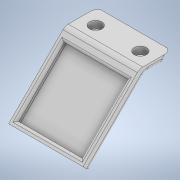
# Autodesk Inventor part: Держатель GPS
Saved by Autodesk Inventor 2022 (Build 260153000, 153)
## iProperties
Created: 2022-05-03
Part Number: Держатель GPS
Material: Типовые
Document SubType Name: Modeling
Designer: Кочетов.А.И.
Density: 1 g/cm^3
Appearance: По умолчанию
Author: Кочетов.А.И.
Autodesk Inventor part; units mm, degrees
ref_plane "YZ Plane" through (0, 0, 0) normal (1, 0, 0) x (0, 1, 0)
ref_plane "XZ Plane" through (0, 0, 0) normal (0, 1, 0) x (-1, 0, 0)
sketch "Эскиз4" plane through (0, 0, 0) normal (0, 1, 0) x (-1, 0, 0)
  line L0 (15, 10) -> (-15, 10)
  line L1 (-15, 10) -> (-15, -10)
  line L2 (-15, -10) -> (15, -10)
  line L3 (15, -10) -> (15, 10)
  line L4 (15, 10) -> (-15, -10) construction
  line L5 (-15, 10) -> (15, -10) construction
  line L6 (15, 0) -> (-15, 0) construction
  line L7 (15, 0) -> (-15, 0)
  point P0 (0, 0)
  dimension "d13" = 30
  dimension "d32" = 20
  constraints: 16 end point, 4 midpoint, 2 parallel, 2 perpendicular, 1 horizontal
  measures "d13" distance of L1.end L2.end
  measures "d32" distance of L0.end L1.end
extrude "Выдавливание4" add sketch "Эскиз4" along normal blind 3 contours L3 L2 L1 L7
ref_plane "РабПлоскость2" through (-15, 0, 0) normal (0, -0.7071068, -0.7071068) x (1, 0, 0)
sketch "Эскиз5" plane through (-15, 0, 0) normal (0, 0, 1) x (1, 0, 0)
  line L0 (0, 0) -> (30, 0) projected
  line L1 (30, 0) -> (30, 3) projected
  line L2 (0, 3) -> (30, 3) projected
  line L3 (0, 0) -> (0, 3) projected
  point P0 (15, 0)
extrude "Выдавливание5" add sketch "Эскиз5" along normal blind 2
sketch "Эскиз6" plane through (-15, 0, 0) normal (0, -0.7071068, -0.7071068) x (1, 0, 0)
  line L0 (0, -7.0711) -> (0, 1.4142) projected
  line L1 (0, 0) -> (30, 0)
  line L2 (30, 0) -> (30, 30)
  line L3 (30, 30) -> (0, 30)
  line L4 (0, 30) -> (0, 0)
  line L5 (30, -7.0711) -> (30, 1.4142) projected
  line L6 (30, -7.0711) -> (30, -9.1924) projected
  line L7 (30, -9.1924) -> (30, -0.7071) projected
  line L8 (30, 1.4142) -> (30, -0.7071) projected
  line L9 (2, 28) -> (28, 28)
  line L10 (28, 28) -> (28, 2)
  line L11 (28, 2) -> (2, 2)
  line L12 (2, 2) -> (2, 28)
  point P0 (15, 0)
  point P1 (0, 1.4142)
  dimension "d19" = 30
  dimension "d20" = 2
  dimension "d21" = 2
  dimension "d22" = 2
  dimension "d23" = 26
  constraints: 16 end point, 4 parallel, 2 horizontal, 2 perpendicular, 2 point on line, 1 midpoint
  measures "d19" distance between parallel lines of L3 L1
  measures "d20" distance between parallel lines of L3 L9
  measures "d21" distance between parallel lines of L2 L10
  measures "d22" distance between parallel lines of L4 L12
  measures "d23" distance between parallel lines of L9 L11
extrude "Выдавливание6" add sketch "Эскиз6" against normal blind 2
sketch "Эскиз7" plane through (-15, 0, 0) normal (0, -0.7071068, -0.7071068) x (-1, 0, 0)
  line L0 (0, -30) -> (0, 0) projected
  line L1 (-30, 0) -> (0, 0) projected
  line L2 (-30, 0) -> (-30, -30) projected
  line L3 (-30, -30) -> (0, -30) projected
  line L4 (-2, -28) -> (-28, -28) projected
  line L5 (-28, -28) -> (-28, -2) projected
  line L6 (-28, -2) -> (-2, -2) projected
  line L7 (-2, -2) -> (-2, -28) projected
  point P0 (-15, 0)
extrude "Выдавливание7" add sketch "Эскиз7" along normal blind 2 contours L3 L2 L1 L0 | L4 L5 L6 L7
sketch "Эскиз8" plane through (15, 0, 0) normal (0, 0.7071068, -0.7071068) x (-1, 0, 0)
  line L0 (0, 0) -> (30, 0) projected
  line L1 (0, 0) -> (0, -2) projected
  line L2 (30, -2) -> (0, -2) projected
  line L3 (30, 0) -> (30, -2) projected
  point P0 (15, 0)
extrude "Выдавливание8" add sketch "Эскиз8" against normal up to surface surface through (0, 0, -5) normal (0, 1, 0)
sketch "Эскиз9" plane through (15, 0, -10) normal (1, 0, 0) x (0, 0, -1)
  line L0 (-12, 0.8284) -> (-12, 3) projected
  line L1 (-12, 0.8284) -> (-9.8284, 3)
  line L2 (0, 3) -> (-12, 3) projected
  line L3 (-32.6274, -19.799) -> (-12, 0.8284) projected
  point P0 (-10, 0)
  constraints: 2 end point, 2 point on line
extrude "Выдавливание9" cut sketch "Эскиз9" against normal through all
sketch "Эскиз10" plane through (0, 0, 0) normal (0, -1, 0) x (1, 0, 0)
  circle A0 centre (9, -6.5) radius 2.5
  circle A1 centre (-9, -6.5) radius 2.5
  line L0 (0, 4.8636) -> (0, -12.9968) construction
  line L1 (15, -10) -> (-15, -10) construction
  point P0 (0, 0)
  dimension "d33" = 5
  dimension "d34" = 18
  dimension "d35" = 3.5
  constraints: 2 centre point, 2 end point, 1 equal radius, 1 point on line, 1 symmetric about line, 1 vertical
  measures "d33" diameter of A0
  measures "d34" distance of A1.centre A0.centre
  measures "d35" distance from line of L1 A0.centre
extrude "Выдавливание10" cut sketch "Эскиз10" against normal through all
fillet "Сопряжение1" radius 3 1 edges at (0, 3, -0.1716)
fillet "Сопряжение2" radius 2 1 edges at (0, 0, -2.8284)
fillet "Сопряжение3" radius 1 4 edges at (0, 0, 2.8284) (13, -9.1924, 12.0208) (0, -18.3848, 21.2132) (-13, -9.1924, 12.0208)
sketch "Эскиз11" plane through (-15, 0, -10) normal (-1, 0, 0) x (0, 0, 1)
  line L0 (0, 0) -> (-3, 3)
  line L1 (29.799, -22.6274) -> (7.7574, -0.5858) projected
  arc A0 (10.7071, 2.1213) -> (8.5858, 3) centre (8.5858, 0) ccw projected
  line L2 (0, 3) -> (8.5858, 3) projected
  line L3 (0, 0) -> (0, 3) projected
  line L4 (0, 0) -> (6.3431, 0) projected
  arc A1 (7.7574, -0.5858) -> (6.3431, 0) centre (6.3431, -2) ccw projected
  line L5 (29.799, -22.6274) -> (7.7574, -0.5858) projected
  line L6 (29.799, -22.6274) -> (32.6274, -19.799) projected
  line L7 (32.6274, -19.799) -> (10.7071, 2.1213) projected
  line L8 (0, 3) -> (-3, 3)
  point P0 (10, 0)
  constraints: 5 end point, 1 horizontal, 1 parallel
extrude "Выдавливание11" add sketch "Эскиз11" against normal up to surface (30 mm away) contours L0 L8 L3
fillet "Сопряжение4" radius 2 1 edges at (0, 0, -10)
fillet "Сопряжение5" radius 2 11 edges at (0, -22.6274, 19.799) (15, -0.1522, -2.8915) (15, 0, -6.4142) (15, 0.1522, -9.9369) (15, 1.7929, -11.7929) (15, -11.6066, 8.7782) (-15, -0.1522, -2.8915) (-15, 0, -6.4142) (-15, 0.1522, -9.9369) (-15, 1.7929, -11.7929) (-15, -11.6066, 8.7782)
